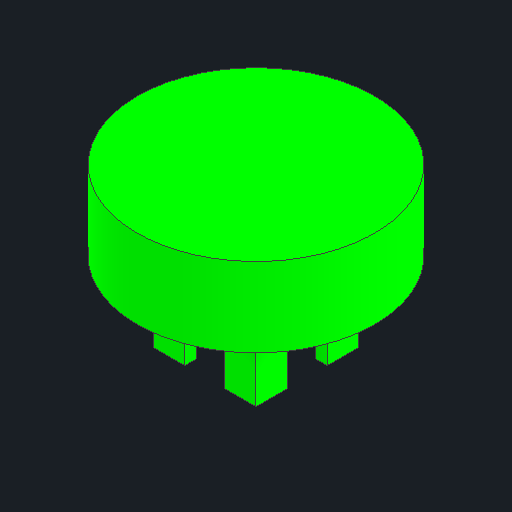
# Autodesk Inventor part: Inflate_Button
Saved by Autodesk Inventor 2026.2 (Build 302298000, 298)
## iProperties
Created: 2026-04-03
Part Number: Inflate_Button
Material: Default New Material
Document SubType Name: Modeling
Designer: vckot
Density: 1 g/cm^3
Appearance: Generic
Author: vckot
Autodesk Inventor part; units mm, degrees
ref_plane "YZ Plane" through (0, 0, 0) normal (1, 0, 0) x (0, 1, 0)
ref_plane "XZ Plane" through (0, 0, 0) normal (0, 1, 0) x (-1, 0, 0)
ref_plane "XY Plane" through (0, 0, 0) normal (0, 0, 1) x (1, 0, 0)
sketch "Sketch1" plane through (0, 0, 0) normal (0, 1, 0) x (-1, 0, 0)
  circle A0 centre (0, 0) radius 7.5
  line L0 (-3.25, 3.25) -> (3.25, 3.25)
  line L1 (3.25, 3.25) -> (3.25, -3.25)
  line L2 (3.25, -3.25) -> (-3.25, -3.25)
  line L3 (-3.25, -3.25) -> (-3.25, 3.25)
  line L4 (-3.25, 3.25) -> (3.25, -3.25) construction
  line L5 (3.25, 3.25) -> (-3.25, -3.25) construction
  line L6 (-2.5, 2.5) -> (2.5, 2.5)
  line L7 (2.5, 2.5) -> (2.5, -2.5)
  line L8 (2.5, -2.5) -> (-2.5, -2.5)
  line L9 (-2.5, -2.5) -> (-2.5, 2.5)
  line L10 (-2.5, 2.5) -> (2.5, -2.5) construction
  line L11 (2.5, 2.5) -> (-2.5, -2.5) construction
  line L12 (2.5, 1.25) -> (3.25, 1.25)
  line L13 (2.5, -1.25) -> (3.25, -1.25)
  line L14 (1.25, 2.5) -> (1.25, 3.25)
  line L15 (-1.25, 3.25) -> (-1.25, 2.5)
  line L16 (3.25, 0) -> (-3.25, 0) construction
  line L17 (0, 3.25) -> (0, -3.25) construction
  line L18 (-2.5, 1.25) -> (-3.25, 1.25)
  line L19 (-2.5, -1.25) -> (-3.25, -1.25)
  line L20 (1.25, -2.5) -> (1.25, -3.25)
  line L21 (-1.25, -3.25) -> (-1.25, -2.5)
  point P0 (2.875, -1.25)
  point P1 (2.875, 1.25)
  point P2 (-1.25, 2.875)
  point P3 (1.25, 2.875)
  dimension "d0" = 15
  dimension "d1" = 6.5
  dimension "d2" = 6.5
  dimension "d3" = 5
  dimension "d4" = 2.5
  dimension "d5" = 1.25
  dimension "d6" = 2.5
  dimension "d7" = 1.25
  constraints: 44 end point, 12 midpoint, 9 point on line, 8 symmetric about line, 6 parallel, 4 perpendicular, 2 horizontal, 1 centre point, 1 coincident
  measures "d0" diameter of A0
  measures "d1" distance of L1.end L2.end
  measures "d2" distance of L0.end L1.end
  measures "d3" distance of L7.end L8.end
  measures "d4" distance of point (2.875, -1.25) point (2.875, 1.25)
  measures "d5" distance from line of L12 A0.centre
  measures "d6" distance of point (-1.25, 2.875) point (1.25, 2.875)
  measures "d7" distance from line of L14 A0.centre
extrude "Extrusion1" add sketch "Sketch1" along normal blind 5 contours A0 | L0 L15 L6 L9 L18 L3 | L0 L14 L6 L15 | L18 L9 L19 L3 | L0 L1 L12 L7 L6 L14 | L6 L7 L8 L9 | L19 L9 L8 L21 L2 L3 | L1 L13 L7 L12 | L21 L8 L20 L2 | L1 L2 L20 L8 L7 L13
extrude "Extrusion2" add sketch "Sketch1" against normal blind 5 contours L0 L15 L6 L9 L18 L3 | L0 L1 L12 L7 L6 L14 | L19 L9 L8 L21 L2 L3 | L1 L2 L20 L8 L7 L13
equation "\"d5\" = 0.5 * d4"
equation "\"d7\" = 0.5 * d6"
body "Solid1"
